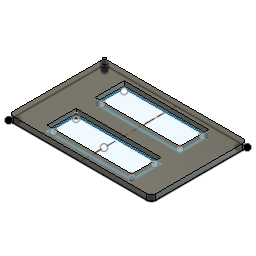
2xIbidi_8ChamberSlide-PlateInsert_ v1 (Autodesk Fusion 360 design; units mm, degrees)
Autodesk Fusion 360 part; units mm, degrees
sketch "Sketch1" plane through (0, 0, 0) normal (0, 1, 0) x (1, 0, 0)
  line L0 (5, -15) -> (56.3866, -15)
  line L1 (56.3866, -15) -> (56.3866, -37.4714)
  line L2 (56.3866, -37.4714) -> (5, -37.4714)
  line L3 (5, -37.4714) -> (5, -15)
  constraint horizontal L0
  constraint vertical L1
  constraint horizontal L2
  constraint vertical L3
sketch "Sketch2" plane through (0, 0, 0) normal (0, 1, 0) x (1, 0, 0)
  line L0 (4, 0) -> (124, 0)
  line L1 (128, -4) -> (128, -82)
  line L2 (124, -86) -> (4, -86)
  line L3 (0, -82) -> (0, -4)
  arc A0 (4, 0) -> (0, -4) centre (4, -4) ccw
  arc A1 (128, -4) -> (124, 0) centre (124, -4) ccw
  arc A2 (0, -82) -> (4, -86) centre (4, -82) ccw
  arc A3 (124, -86) -> (128, -82) centre (124, -82) ccw
  line L4 (64, -86) -> (64, 0) construction
  line L5 (64, -43) -> (64, -21.5) construction
  line L6 (64, -21.5) -> (64, -8.5) construction
  line L7 (64, -8.5) -> (26, -8.5) construction
  line L8 (26, -8.5) -> (102, -8.5)
  line L9 (102, -8.5) -> (102, -34.5)
  line L10 (102, -34.5) -> (26, -34.5)
  line L11 (26, -34.5) -> (26, -8.5)
  line L12 (26, -8.5) -> (27, -8.5) construction
  line L13 (27, -8.5) -> (27, -9.5) construction
  line L14 (29, -9.5) -> (99, -9.5)
  line L15 (101, -11.5) -> (101, -31.5)
  line L16 (99, -33.5) -> (29, -33.5)
  line L17 (27, -31.5) -> (27, -11.5)
  line L18 (64, -64.5) -> (64, -77.5) construction
  line L19 (64, -77.5) -> (26, -77.5) construction
  line L20 (26, -77.5) -> (102, -77.5)
  line L21 (102, -77.5) -> (102, -51.5)
  line L22 (102, -51.5) -> (26, -51.5)
  line L23 (26, -51.5) -> (26, -77.5)
  line L24 (26, -77.5) -> (26, -76.5)
  line L25 (26, -76.5) -> (27, -76.5)
  line L26 (29, -76.5) -> (99, -76.5)
  line L27 (101, -74.5) -> (101, -54.5)
  line L28 (99, -52.5) -> (29, -52.5)
  line L29 (27, -54.5) -> (27, -74.5)
  arc A4 (29, -52.5) -> (27, -54.5) centre (29, -54.5) ccw
  arc A5 (27, -74.5) -> (29, -76.5) centre (29, -74.5) ccw
  arc A6 (101, -54.5) -> (99, -52.5) centre (99, -54.5) ccw
  arc A7 (99, -76.5) -> (101, -74.5) centre (99, -74.5) ccw
  arc A8 (29, -9.5) -> (27, -11.5) centre (29, -11.5) ccw
  arc A9 (27, -31.5) -> (29, -33.5) centre (29, -31.5) ccw
  arc A10 (99, -33.5) -> (101, -31.5) centre (99, -31.5) ccw
  arc A11 (101, -11.5) -> (99, -9.5) centre (99, -11.5) ccw
  circle A12 centre (4, -4) radius 1.5
  point P0 (128, 0)
  point P1 (0, -86)
  point P2 (101, -9.5)
  point P3 (27, -33.5)
  point P4 (101, -76.5)
  point P5 (27, -52.5)
  dimension "d3" = 128
  dimension "d4" = 86
  dimension "d5" = 4
  dimension "d6" = 4
  dimension "d7" = 4
  dimension "d8" = 4
  dimension "d12" = 76
  dimension "d13" = 26
  dimension "d14" = 1
  dimension "d15" = 74
  dimension "d16" = 24
  dimension "d20" = 76
  dimension "d21" = 26
  dimension "d22" = 74
  dimension "d23" = 24
  dimension "d24" = 2
  dimension "d25" = 2
  dimension "d26" = 2
  dimension "d27" = 2
  dimension "d28" = 2
  dimension "d29" = 2
  dimension "d30" = 2
  dimension "d31" = 2
  dimension "d32" = 3
  constraint horizontal L0
  constraint vertical L1
  constraint horizontal L2
  constraint vertical L3
  constraint coincident origin L0
  constraint coincident origin L3
  constraint tangent L0 A0
  constraint tangent L3 A0
  constraint coincident P0 L0
  constraint coincident P0 L1
  constraint tangent L0 A1
  constraint tangent L1 A1
  constraint coincident P1 L2
  constraint coincident P1 L3
  constraint tangent L2 A2
  constraint tangent L3 A2
  constraint tangent L1 A3
  constraint tangent L2 A3
  constraint midpoint L2 L4.start
  constraint midpoint L0 L4.end
  constraint midpoint L4 L5.start
  constraint parallel L4 L6
  constraint perpendicular L4 L7
  constraint horizontal L8
  constraint vertical L9
  constraint horizontal L10
  constraint vertical L11
  constraint horizontal L12
  constraint perpendicular L12 L13
  constraint horizontal L14
  constraint vertical L15
  constraint horizontal L16
  constraint vertical L17
  constraint parallel L4 L18
  constraint perpendicular L4 L19
  constraint horizontal L20
  constraint vertical L21
  constraint horizontal L22
  constraint vertical L23
  constraint coincident L23 L24.end
  constraint perpendicular L20 L24
  constraint perpendicular L24 L25
  constraint horizontal L26
  constraint vertical L27
  constraint horizontal L28
  constraint vertical L29
  constraint coincident P5 L28
  constraint coincident P5 L29
  constraint tangent L28 A4
  constraint tangent L29 A4
  constraint coincident L25.end L26
  constraint coincident L25.end L29
  constraint tangent L26 A5
  constraint tangent L29 A5
  constraint tangent L27 A6
  constraint tangent L28 A6
  constraint coincident P4 L26
  constraint coincident P4 L27
  constraint tangent L26 A7
  constraint tangent L27 A7
  constraint coincident L13.end L17
  constraint coincident L13.end L14
  constraint tangent L17 A8
  constraint tangent L14 A8
  constraint coincident P3 L16
  constraint coincident P3 L17
  constraint tangent L16 A9
  constraint tangent L17 A9
  constraint tangent L15 A10
  constraint tangent L16 A10
  constraint coincident P2 L14
  constraint coincident P2 L15
  constraint tangent L14 A11
  constraint tangent L15 A11
  constraint concentric A0 A12
  measures "d3" distance of origin P0
  measures "d4" distance of origin P1
  measures "d5" radius of A0
  measures "d6" radius of A1
  measures "d7" radius of A2
  measures "d8" radius of A3
  measures "d12" distance of L7.end L8.end
  measures "d13" distance of L7.end L10.end
  measures "d14" distance of L7.end L12.end
  measures "d15" distance of L13.end P2
  measures "d16" distance of L13.end P3
  measures "d20" distance of L19.end L20.end
  measures "d21" distance of L19.end L22.end
  measures "d22" distance of L25.end P4
  measures "d23" distance of L25.end P5
  measures "d24" radius of A4
  measures "d25" radius of A5
  measures "d26" radius of A6
  measures "d27" radius of A7
  measures "d28" radius of A8
  measures "d29" radius of A9
  measures "d30" radius of A10
  measures "d31" radius of A11
  measures "d32" diameter of A12
extrude "Extrude2" add sketch "Sketch2" along normal blind 5 contours L0 L1 L2 L3 A0 A1 A2 A3
extrude "Extrude3" add sketch "Sketch2" along normal blind 0.5 contours L8 L9 L10 L11
extrude "Extrude4" add 1 faces at (52.3333, 0.5, 34.1667) along direction (0, 1, 0) blind 0.5
extrude "Extrude5" add sketch "Sketch2" along normal blind 1 contours L20 L21 L22 L23 L24
extrude "Extrude6" add sketch "Sketch2" along normal blind 12 contours A12
extrude "Extrude7" cut 1 faces at (3.584, 12, 3.3234) along direction (0, -1, 0) blind 5
extrude "Extrude8" add 1 faces at (3.584, 7, 3.3234) along direction (0, 1, 0) blind 2
